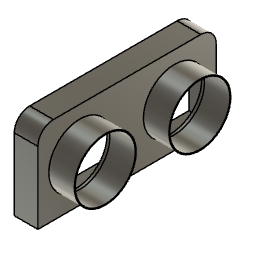
Ultrasonic_Sensor_Enclosure (Autodesk Fusion 360 design; units mm, degrees)
Autodesk Fusion 360 part; units mm, degrees
sketch "Sketch1" plane through (0, 0, 0) normal (1, 0, 0) x (0, 1, 0)
  line L0 (0, 0) -> (49, 0)
  line L1 (49, 0) -> (49, 19.75)
  line L2 (44.75, 24) -> (4.25, 24)
  line L3 (0, 19.75) -> (0, 0)
  arc A0 (49, 19.75) -> (44.75, 24) centre (44.75, 19.75) ccw
  arc A1 (49, 19.75) -> (44.75, 24) centre (44.75, 19.75) ccw
  arc A2 (4.25, 24) -> (0, 19.75) centre (4.25, 19.75) ccw
  circle A3 centre (11.5, 12) radius 8.5
  circle A4 centre (37.5, 12) radius 8.5
  dimension "d1" = 49
  dimension "d11" = 17
  dimension "d12" = 17
  dimension "d13" = 11.5
  dimension "d14" = 11.5
  dimension "d16" = 12
  dimension "d17" = 12
  constraint horizontal L0
  constraint vertical L1
  constraint horizontal L2
  constraint vertical L3
  constraint coincident L0.start L3.end
  measures "d1" distance of L0.start L0.end
  measures "d11" diameter of A3
  measures "d12" diameter of A4
  measures "d13" distance of L3 A3.centre
  measures "d14" distance of L1 A4.centre
  measures "d16" distance of L2 A3.centre
  measures "d17" distance of L2 A4.centre
extrude "Extrude1" add sketch "Sketch1" along normal blind 2.5 makes body 1
sketch "Sketch2" plane through (2.5, 0, 0) normal (1, 0, 0) x (0, 1, 0)
  circle A0 centre (37.5, 12) radius 8.5
  circle A1 centre (11.5, 12) radius 8.5
  arc A2 (4.25, 24) -> (0, 19.75) centre (4.25, 19.75) ccw
  line L0 (0, 19.75) -> (0, 0)
  line L1 (0, 0) -> (49, 0)
  line L2 (49, 0) -> (49, 19.75)
  arc A3 (49, 19.75) -> (44.75, 24) centre (44.75, 19.75) ccw
  line L3 (44.75, 24) -> (4.25, 24)
  circle A4 centre (11.5, 12) radius 8.5
  constraint concentric A1 A4
extrude "Extrude2" add sketch "Sketch2" along normal blind 12 separate body contours A1 A4 makes body 2
sketch "Sketch3" plane through (2.5, 0, 0) normal (1, 0, 0) x (0, 1, 0)
  circle A0 centre (37.5, 12) radius 8.5
  circle A1 centre (11.5, 12) radius 8.5
  arc A2 (4.25, 24) -> (0, 19.75) centre (4.25, 19.75) ccw
  line L0 (0, 19.75) -> (0, 0)
  line L1 (0, 0) -> (49, 0)
  line L2 (49, 0) -> (49, 19.75)
  arc A3 (49, 19.75) -> (44.75, 24) centre (44.75, 19.75) ccw
  line L3 (44.75, 24) -> (4.25, 24)
  circle A4 centre (37.5, 12) radius 8.5
  constraint concentric A0 A4
extrude "Extrude3" add sketch "Sketch3" along normal blind 12 separate body contours A0 A4 makes body 3
hole "Hole1" at (14.5, 11.5, 12) direction (-1, 0, 0) diameter 16.5 depth 15 tip angle 118 bodies 2
hole "Hole2" at (14.5, 37.5, 12) direction (-1, 0, 0) diameter 16.5 depth 15 tip angle 118 bodies 3
extrude "Extrude4" add 1 faces at (0, 20.7971, 1.2377) along direction (-1, 0, 0) blind 3.5 on bodies 1 bodies 1
extrude "Extrude5" add 1 faces at (-3.5, 20.7971, 1.2377) along direction (-1, 0, 0) blind 0.5 on bodies 1 bodies 1
sketch "Sketch4" plane through (-4, 0, 0) normal (-1, 0, 0) x (0, -1, 0)
  circle A0 centre (-37.5, 12) radius 8.5
  circle A1 centre (-11.5, 12) radius 8.5
  arc A2 (0, 19.75) -> (-4.25, 24) centre (-4.25, 19.75) ccw
  line L0 (-4.25, 24) -> (-44.75, 24)
  arc A3 (-44.75, 24) -> (-49, 19.75) centre (-44.75, 19.75) ccw
  line L1 (-49, 19.75) -> (-49, 0)
  line L2 (-49, 0) -> (0, 0)
  line L3 (0, 0) -> (0, 19.75)
  line L4 (-48, 1) -> (-1, 1)
  line L5 (-1, 1) -> (-1, 21)
  line L6 (-1, 21) -> (-48, 21)
  line L7 (-48, 21) -> (-48, 1)
  dimension "d34" = 47
  dimension "d35" = 20
  constraint horizontal L4
  constraint vertical L5
  constraint horizontal L6
  constraint vertical L7
  measures "d34" distance of L4.start L4.end
  measures "d35" distance of L4.start L6.end
extrude "Extrude6" cut sketch "Sketch4" against normal blind 5.5 contours L4 L5 L6 L7 bodies 1
sketch "Sketch5" plane through (-4, 0, 0) normal (-1, 0, 0) x (0, -1, 0)
  line L0 (-1, 1) -> (-48, 1)
  line L1 (-48, 1) -> (-48, 21)
  line L2 (-48, 21) -> (-1, 21)
  line L3 (-1, 21) -> (-1, 1)
  arc A0 (0, 19.75) -> (-4.25, 24) centre (-4.25, 19.75) ccw
  line L4 (-4.25, 24) -> (-44.75, 24)
  arc A1 (-44.75, 24) -> (-49, 19.75) centre (-44.75, 19.75) ccw
  line L5 (-49, 19.75) -> (-49, 0)
  line L6 (-49, 0) -> (0, 0)
  line L7 (0, 0) -> (0, 19.75)
  line L8 (-30.5, 23) -> (-18.5, 23)
  line L9 (-18.5, 23) -> (-18.5, 21)
  line L10 (-18.5, 21) -> (-30.5, 21)
  line L11 (-30.5, 21) -> (-30.5, 23)
  dimension "d38" = 12
  dimension "d39" = 2
  dimension "d40" = 18.5
  constraint horizontal L8
  constraint vertical L9
  constraint horizontal L10
  constraint vertical L11
  measures "d38" distance of L8.start L8.end
  measures "d39" distance of L8.start L10.end
  measures "d40" distance of L5 L11
extrude "Extrude7" cut sketch "Sketch5" against normal blind 5.5 contours L2 L8 L9 L10 L11 bodies 1
extrude "Extrude8" cut 1 faces at (14.5, 44.9942, 8.391) along direction (-1, 0, 0) blind 5 on bodies 3 bodies 3
extrude "Extrude9" cut 1 faces at (14.5, 9.6491, 20.1094) along direction (-1, 0, 0) blind 5 on bodies 2 bodies 2
